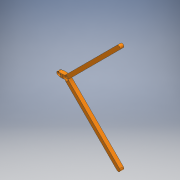
# Autodesk Inventor part: 压缩杆
Saved by Autodesk Inventor 2017 (Build 210142000, 142)
## iProperties
Part Number: 压缩杆
Material: 常规
Document SubType Name: Modeling
Designer: PANDA
Density: 1 g/cm^3
Appearance: 默认
Author: PANDA
Autodesk Inventor part; units mm, degrees
ref_plane "YZ Plane" through (0, 0, 0) normal (1, 0, 0) x (0, 1, 0)
ref_plane "XZ Plane" through (0, 0, 0) normal (0, 1, 0) x (-1, 0, 0)
ref_plane "XY Plane" through (0, 0, 0) normal (0, 0, 1) x (1, 0, 0)
sketch "草图2" plane through (0, 0, 0) normal (0, 1, 0) x (-1, 0, 0)
  line L0 (5, 0) -> (-5, 0) construction
  line L1 (5, 2.5) -> (-5, 2.5)
  line L2 (-5, -2.5) -> (5, -2.5)
  arc A0 (5, -2.5) -> (5, 2.5) centre (5, 0) ccw
  arc A1 (-5, 2.5) -> (-5, -2.5) centre (-5, 0) ccw
  line L3 (5, 0) -> (15, 0) construction
  circle A2 centre (5, 0) radius 2
  circle A3 centre (-5, 0) radius 2
  point P0 (0, 0)
  point P1 (0, 0)
  dimension "d6" = 10
  dimension "d7" = 180
  dimension "d8" = 5
  dimension "d9" = 4
  dimension "d10" = 4
  constraints: 10 end point, 4 centre point, 4 point on circle, 4 tangent, 2 coincident, 2 horizontal, 1 collinear, 1 midpoint, 1 parallel
  measures "d6" distance of L0.start L0.end
  measures "d7" angle of L0 L3
  measures "d8" diameter of A1
  measures "d9" diameter of A2
  measures "d10" diameter of A3
extrude "拉伸1" add sketch "草图2" along normal blind 5
sketch "草图3" plane through (0, 5, 0) normal (0, 1, 0) x (1, 0, 0)
  line L0 (5, 0) -> (75.7107, 70.7107) construction
  line L1 (6.7678, -1.7678) -> (77.4784, 68.9429)
  line L2 (73.9429, 72.4784) -> (3.2322, 1.7678)
  arc A0 (3.2322, 1.7678) -> (6.7678, -1.7678) centre (5, 0) ccw
  arc A1 (77.4784, 68.9429) -> (73.9429, 72.4784) centre (75.7107, 70.7107) ccw
  line L3 (5, 0) -> (105, 0) construction
  line L4 (5, 0) -> (75.7107, -70.7107) construction
  line L5 (3.2322, -1.7678) -> (73.9429, -72.4784)
  line L6 (77.4784, -68.9429) -> (6.7678, 1.7678)
  arc A2 (6.7678, 1.7678) -> (3.2322, -1.7678) centre (5, 0) ccw
  arc A3 (73.9429, -72.4784) -> (77.4784, -68.9429) centre (75.7107, -70.7107) ccw
  line L7 (5, 0) -> (105, 0) construction
  point P0 (0, 0)
  point P1 (40.3553, 35.3553)
  point P2 (40.3553, -35.3553)
  dimension "d13" = 100
  dimension "d14" = 45
  dimension "d15" = 5
  dimension "d16" = 100
  dimension "d17" = 45
  dimension "d18" = 5
  constraints: 20 end point, 8 point on circle, 8 tangent, 4 centre point, 2 equal length, 2 horizontal, 2 midpoint, 2 parallel, 1 perpendicular
  measures "d13" distance of L0.start L0.end
  measures "d14" angle of L3 L0
  measures "d15" diameter of A1
  measures "d16" distance of L0.start L4.end
  measures "d17" angle of L4 L7
  measures "d18" diameter of A3
extrude "拉伸2" add sketch "草图3" against normal blind 5
sketch "草图4" plane through (0, 5, 0) normal (0, 1, 0) x (1, 0, 0)
  circle A0 centre (5, 0) radius 2
  point P0 (0, 0)
  dimension "d21" = 4
  constraints: 1 centre point
  measures "d21" diameter of A0
extrude "拉伸3" cut sketch "草图4" against normal through all
fillet "圆角1" radius 2 4 edges at (3, 0, 0) (3, 5, 0) (-3, 5, 0) (-3, 0, 0)
